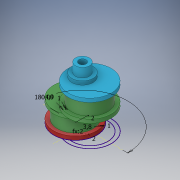
# Autodesk Inventor part: ExcentricShaft
Saved by Autodesk Inventor 2018.3 (Build 223284000, 284)
## iProperties
Created: 2018-07-20
Part Number: ExcentricShaft
Material: Generisch
Document SubType Name: Modeling
Designer: JochenAlt
Density: 1 g/cm^3
Appearance: Türkis
Author: JochenAlt
Autodesk Inventor part; units mm, degrees
ref_plane "YZ Plane" through (0, 0, 0) normal (1, 0, 0) x (0, 1, 0)
ref_plane "XZ Plane" through (0, 0, 0) normal (0, 1, 0) x (-1, 0, 0)
ref_plane "XY Plane" through (0, 0, 0) normal (0, 0, 1) x (1, 0, 0)
sketch "Skizze1" plane through (0, 0, 0) normal (0, 0, 1) x (1, 0, 0)
  line L0 (0, 8.26) -> (0, -8.26) construction
  line L1 (-11.06, 0) -> (11.06, 0) construction
  circle A0 centre (0, 0) radius 1.9
  arc A1 (1.35, -4.8567) -> (1.35, 4.8567) centre (2, 0) ccw
  line L2 (0, -2) -> (0, 0) construction
  line L3 (0, 0) -> (2, 0) construction
  arc A2 (-1.35, 4.8567) -> (-1.35, -4.8567) centre (-2, 0) ccw
  arc A3 (0, -4.4733) -> (0, 4.4733) centre (-2, 0) ccw
  arc A4 (0, 4.4733) -> (0, -4.4733) centre (2, 0) ccw
  line L4 (0, 0) -> (-6.4757, 0) construction
  circle A5 centre (0, 0) radius 2.9
  arc A6 (0, 5.5507) -> (-1.35, 4.8567) centre (2, 0) ccw
  arc A7 (1.35, 4.8567) -> (0, 4.4733) centre (2, 0) ccw
  arc A8 (-1.35, 4.8567) -> (-1.35, -4.8567) centre (2, 0) ccw
  arc A9 (0, -5.5507) -> (0, 5.5507) centre (2, 0) ccw
  arc A10 (-1.35, -4.8567) -> (0, -5.5507) centre (2, 0) ccw
  arc A11 (0, -4.4733) -> (1.35, -4.8567) centre (2, 0) ccw
  arc A12 (-1.35, -4.8567) -> (0, -4.4733) centre (-2, 0) ccw
  arc A13 (0, -5.5507) -> (1.35, -4.8567) centre (-2, 0) ccw
  arc A14 (1.35, -4.8567) -> (1.35, 4.8567) centre (-2, 0) ccw
  arc A15 (0, 5.5507) -> (0, -5.5507) centre (-2, 0) ccw
  arc A16 (0, 4.4733) -> (-1.35, 4.8567) centre (-2, 0) ccw
  arc A17 (1.35, 4.8567) -> (0, 5.5507) centre (-2, 0) ccw
  circle A18 centre (0, 0) radius 1
  dimension "d0" = 3.8
  dimension "d1" = 2
  dimension "d13" = 4.9
  dimension "d16" = 180
  dimension "d17" = 2
  dimension "d18" = 1
  dimension "d26" = 1
  dimension "d27" = 2
  constraints: 34 point on circle, 19 centre point, 14 equal radius, 6 end point, 5 coincident, 2 collinear, 2 concentric, 2 point on line, 1 perpendicular
  measures "d0" diameter of A0
  measures "d1" distance of point (0, 0) A2.centre
  measures "d13" radius of A2
  measures "d16" angle of L4 L1
  measures "d17" distance of point (0, 0) L3.end
  measures "d18" radial gap between concentric circles of A5 A0
  measures "d26" radial gap between concentric circles of A15 A2
  measures "d27" diameter of A18
extrude "Extrusion10" add sketch "Skizze1" along normal blind 1 contours A0 | A13 A10 A12 A11 | A11 A3 A7 A14 | A7 A16 A6 A17 | A4 A5 A3 | A12 A8 A16 A4 | A15 A6 A2 A10 | A3 A5 A4 | A5 | A2 A8
extrude "Extrusion2" add sketch "Skizze1" along normal blind 4 from surface at 1 separate body contours A0 | A4 A5 A3 | A12 A8 A16 A4 | A3 A5 A4 | A5 | A2 A8
extrude "Extrusion8" add sketch "Skizze1" along normal blind 1 from surface at 5 contours A0 | A13 A10 A12 A11 | A11 A3 A7 A14 | A7 A16 A6 A17 | A4 A5 A3 | A12 A8 A16 A4 | A15 A6 A2 A10 | A3 A5 A4 | A5 | A2 A8 bodies 2
extrude "Extrusion9" add sketch "Skizze1" along normal blind 1 from surface at 6 contours A0 | A14 A1 | A13 A10 A12 A11 | A1 A17 A9 A13 | A11 A3 A7 A14 | A7 A16 A6 A17 | A4 A5 A3 | A12 A8 A16 A4 | A3 A5 A4 | A5 bodies 2
extrude "Extrusion4" add sketch "Skizze1" along normal blind 4 from surface at 7 contours A0 | A14 A1 | A11 A3 A7 A14 | A4 A5 A3 | A3 A5 A4 | A5 bodies 2
extrude "Extrusion11" add sketch "Skizze1" along normal blind 1 from surface at 11 separate body contours A0 | A14 A1 | A13 A10 A12 A11 | A1 A17 A9 A13 | A11 A3 A7 A14 | A7 A16 A6 A17 | A4 A5 A3 | A12 A8 A16 A4 | A3 A5 A4 | A5
extrude "Extrusion7" add sketch "Skizze1" along normal blind 1 from surface at 12 contours A0 | A5 bodies 3
extrude "Extrusion5" add sketch "Skizze1" along normal blind 2.5 from surface at 13 contours A0 bodies 3
equation "\"d17\" = d1"
